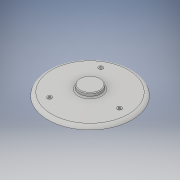
# Autodesk Inventor part: Alojamento do Sensor de Temperatura e Umidade - tampa
Saved by Autodesk Inventor 2019.4 (Build 234330000, 330)
## iProperties
Created: 2021-02-17
Part Number: Alojamento do Sensor de Temperatura e Umidade - tampa
Material: Genérico
Document SubType Name: Modeling
Designer: Lattes
Density: 1 g/cm^3
Appearance: Padrão
Author: Lattes
Autodesk Inventor part; units mm, degrees
ref_plane "YZ Plane" through (0, 0, 0) normal (1, 0, 0) x (0, 1, 0)
ref_plane "XZ Plane" through (0, 0, 0) normal (0, 1, 0) x (-1, 0, 0)
ref_plane "XY Plane" through (0, 0, 0) normal (0, 0, 1) x (1, 0, 0)
sketch "Esboço1" plane through (0, 0, 0) normal (0, 0, 1) x (1, 0, 0)
  line L0 (0, 14) -> (14, 14)
  line L1 (15, 13) -> (15, 9.8301)
  line L2 (16.8229, 7.838) -> (54.5312, 4.4861)
  line L3 (0.6, 13.4) -> (13.4, 13.4)
  line L4 (14.4, 12.4) -> (14.4, 9.2811)
  line L5 (16.2229, 7.2889) -> (53.9312, 3.9371)
  line L6 (0.6, 13.4) -> (0, 13.4)
  line L7 (0, 14) -> (0, 13.4)
  line L8 (0, 0) -> (0, 5.451)
  arc A0 (59.0428, 0) -> (53.9312, 3.9371) centre (53.4, -2.0394) ccw
  arc A1 (59.812, 0) -> (54.5312, 4.4861) centre (54, -1.4903) ccw
  line L9 (59.812, 0) -> (59.0428, 0)
  arc A2 (15, 9.8301) -> (16.8229, 7.838) centre (17, 9.8301) ccw
  arc A3 (14.4, 9.2811) -> (16.2229, 7.2889) centre (16.4, 9.2811) ccw
  arc A4 (14.4, 12.4) -> (13.4, 13.4) centre (13.4, 12.4) ccw
  arc A5 (15, 13) -> (14, 14) centre (14, 13) ccw
  point P0 (60, 4)
  point P1 (15, 14)
  point P2 (15, 8)
  dimension "d4" = 15
  dimension "d5" = 6
  dimension "d7" = 6
  dimension "d8" = 2
  dimension "d9" = 1
  constraints: 20 end point, 12 point on circle, 10 tangent, 6 centre point, 6 point on line, 3 equal radius, 2 horizontal, 2 perpendicular, 1 vertical, 2 other
  measures "d4" distance of L0.start point (15, 14)
  measures "d5" distance of point (15, 14) point (15, 8)
  measures "d7" radius of A0
  measures "d8" radius of A2
  measures "d9" radius of A4
revolve "Revolução1" add sketch "Esboço1" angle 360 about axis through (0, 0, 0) along (0, 1, 0)
sketch "Esboço2" plane through (0, 14, 0) normal (0, 1, 0) x (1, 0, 0)
  line L0 (0, 0) -> (42, 0)
  circle A0 centre (42, 0) radius 1.5
  dimension "d11" = 42
  dimension "d12" = 3
  constraints: 2 end point, 1 centre point, 1 coincident, 1 horizontal
  measures "d11" distance of L0.start L0.end
  measures "d12" diameter of A0
extrude "Extrusão1" cut sketch "Esboço2" against normal blind 20
pattern_circular "Padrão circular1" count 3 over 360 about axis through (0, 6.162, 0) along (0, -1, 0) of "Extrusão1"
ref_plane "Plano de trabalho1" through (0, 6, 0) normal (0, 1, 0) x (1, 0, 0)
sketch "Esboço4" plane through (0, 6, 0) normal (0, 1, 0) x (1, 0, 0)
  line L0 (0, 0) -> (42, 0)
  circle A0 centre (42, 0) radius 1.5
  circle A1 centre (42, 0) radius 3
  dimension "d21" = 42
  dimension "d22" = 3
  dimension "d23" = 6
  constraints: 2 centre point, 2 coincident, 2 end point, 1 horizontal
  measures "d21" distance of L0.start L0.end
  measures "d22" diameter of A0
  measures "d23" diameter of A1
extrude "Extrusão2" add sketch "Esboço4" against normal blind 3
pattern_circular "Padrão circular2" count 3 over 360 about axis through (0, 5.613, 0) along (0, -1, 0) of "Extrusão2"
